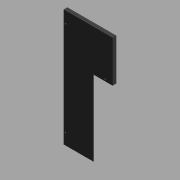
# Autodesk Inventor part: box_front_left
Saved by Autodesk Inventor 2019 (Build 230136000, 136)
## iProperties
Part Number: box_front_left
Material: Generic
Document SubType Name: Modeling
Designer: Javi
Appearance: Default
Author: Javi
Autodesk Inventor part; units mm, degrees
ref_plane "YZ Plane" through (0, 0, 0) normal (1, 0, 0) x (0, 1, 0)
ref_plane "XZ Plane" through (0, 0, 0) normal (0, 1, 0) x (-1, 0, 0)
ref_plane "XY Plane" through (0, 0, 0) normal (0, 0, 1) x (1, 0, 0)
sketch "Sketch1" plane through (0, 0, 0) normal (0, 1, 0) x (-1, 0, 0)
  line L0 (0, 0) -> (-80, 0)
  line L1 (-80, 0) -> (-80, -10)
  line L2 (-80, -10) -> (0, -10)
  line L3 (0, -10) -> (0, 0)
  arc A0 (-62.6378, -10) -> (-80, 0) centre (-130, -106.8831) ccw
  dimension "d1" = 10
  dimension "d2" = 118
  dimension "d3" = 80
  dimension "d4" = 50
  constraints: 8 end point, 2 parallel, 2 point on circle, 1 centre point, 1 horizontal, 1 perpendicular, 1 point on line
  measures "d1" distance of L1.end L0.end
  measures "d2" radius of A0
  measures "d3" distance between parallel lines of L3 L1
  measures "d4" distance from line of L1 A0.centre
extrude "Extrusion1" add sketch "Sketch1" along normal blind 200 contours L3 L2 A0 L0
sketch "Sketch4" plane through (0, 200, 0) normal (0, 1, 0) x (1, 0, 0)
  line L0 (0, 0) -> (130, 0)
  line L1 (130, 0) -> (130, 10)
  line L2 (130, 10) -> (0, 10)
  line L3 (0, 10) -> (0, 0)
  dimension "d24" = 130
  dimension "d25" = 10
  constraints: 8 end point, 2 parallel, 1 horizontal, 1 perpendicular
  measures "d24" distance of L2.end L1.end
  measures "d25" distance of L1.end L0.end
sketch "Sketch3" plane through (0, 0, 0) normal (0, -1, 0) x (1, 0, 0)
  circle A0 centre (30, -5) radius 2
  line L0 (0, 0) -> (80, 0) projected
  line L1 (0, -10) -> (0, 0) projected
  dimension "d19" = 4
  dimension "d20" = 5
  dimension "d21" = 30
  constraints: 1 centre point
  measures "d19" diameter of A0
  measures "d20" distance from line of L0 A0.centre
  measures "d21" distance from line of L1 A0.centre
extrude "Extrusion3" cut sketch "Sketch3" against normal blind 20
sketch "Sketch2" plane through (0, 0, 0) normal (0, 0, 1) x (1, 0, 0)
  circle A0 centre (5, 30) radius 2
  line L0 (0, 0) -> (0, 200) projected
  line L1 (0, 0) -> (80, 0) projected
  circle A1 centre (5, 280) radius 2
  dimension "d7" = 4
  dimension "d8" = 5
  dimension "d9" = 30
  dimension "d12" = 250
  constraints: 2 centre point, 1 vertical, 2 other
  measures "d7" diameter of A0
  measures "d8" distance from line of L0 A0.centre
  measures "d9" distance from line of L1 A0.centre
  measures "d12" distance of A0.centre A1.centre
extrude "Extrusion4" add sketch "Sketch4" along normal blind 110
extrude "Extrusion5" cut sketch "Sketch2" against normal through all
sketch "Sketch5" plane through (0, 0, 0) normal (0, 0, 1) x (1, 0, 0)
  circle A0 centre (110, 205) radius 2
  line L0 (130, 200) -> (130, 310) projected
  line L1 (80, 200) -> (130, 200) projected
  point P0 (0, 0)
  dimension "d30" = 4
  dimension "d31" = 20
  dimension "d32" = 5
  constraints: 1 centre point
  measures "d30" diameter of A0
  measures "d31" distance from line of L0 A0.centre
  measures "d32" distance from line of L1 A0.centre
extrude "Extrusion6" cut sketch "Sketch5" against normal through all
equation "\"d30\" = screws"
equation "\"screws\" = 4"
body "Solid1"
